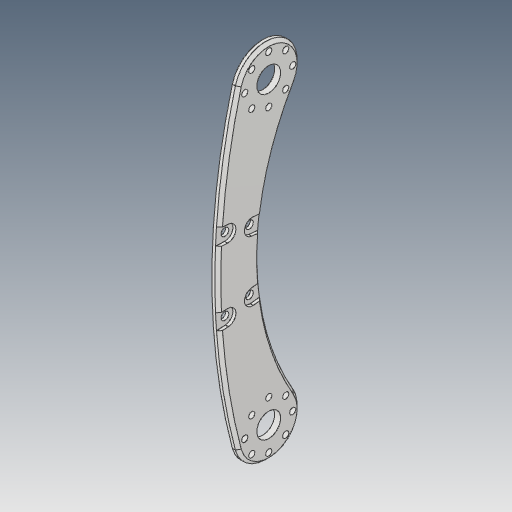
# Autodesk Inventor part: side_frame
Saved by Autodesk Inventor 2019.4 (Build 234330000, 330)
## iProperties
Created: 2018-08-09
Part Number: side_frame
Material: アルミニウム 6061
Document SubType Name: Modeling
Designer: student
Density: 2.7 g/cm^3
Appearance: 滑らか - 白
Mass: 9.43005 g
Surface Area: 44.7876 cm^2
Volume: 3.49261 cm^3
Author: student
Autodesk Inventor part; units mm, degrees
ref_plane "YZ Plane" through (0, 0, 0) normal (1, 0, 0) x (0, 1, 0)
ref_plane "XZ Plane" through (0, 0, 0) normal (0, 1, 0) x (-1, 0, 0)
ref_plane "XY Plane" through (0, 0, 0) normal (0, 0, 1) x (1, 0, 0)
sketch "スケッチ1" plane through (0, 0, 0) normal (1, 0, 0) x (0, 1, 0)
  line L0 (-50, 0) -> (50, 0) construction
  circle A0 centre (-50, 0) radius 4
  circle A1 centre (-50, 0) radius 8 construction
  circle A2 centre (-50, 8) radius 1.05
  line L1 (-50, 8) -> (-50, 0) construction
  circle A3 centre (-55.6569, 5.6569) radius 1.05
  circle A4 centre (-58, 0) radius 1.05
  circle A5 centre (-55.6569, -5.6569) radius 1.05
  circle A6 centre (-50, -8) radius 1.05
  circle A7 centre (-44.3431, -5.6569) radius 1.05
  circle A8 centre (-42, 0) radius 1.05
  circle A9 centre (-44.3431, 5.6569) radius 1.05
  arc A10 (-52.6846, 10.151) -> (-44.7153, -9.0731) centre (-50, 0) ccw
  arc A11 (44.7153, -9.0731) -> (-44.7153, -9.0731) centre (0, -85.8426) ccw
  arc A12 (52.6846, 10.151) -> (-52.6846, 10.151) centre (0, -189.0577) ccw
  arc A13 (44.7153, -9.0731) -> (52.6846, 10.151) centre (50, 0) ccw
  circle A14 centre (50, 0) radius 4
  circle A15 centre (50, 0) radius 8 construction
  line L2 (50, 0) -> (50, 8) construction
  circle A16 centre (50, 8) radius 1.05
  circle A17 centre (44.3431, 5.6569) radius 1.05
  circle A18 centre (42, 0) radius 1.05
  circle A19 centre (44.3431, -5.6569) radius 1.05
  circle A20 centre (50, -8) radius 1.05
  circle A21 centre (55.6569, -5.6569) radius 1.05
  circle A22 centre (58, 0) radius 1.05
  circle A23 centre (55.6569, 5.6569) radius 1.05
  line L3 (12.1598, 13.6356) -> (10.1472, 5.4377) construction
  circle A24 centre (12.1598, 13.6356) radius 1.3
  circle A25 centre (10.1472, 5.4377) radius 1.3
  circle A26 centre (12.1598, 13.6356) radius 3 construction
  circle A27 centre (10.1472, 5.4377) radius 3 construction
  circle A28 centre (-12.1598, 13.6356) radius 1.3
  circle A29 centre (-10.1472, 5.4377) radius 1.3
  line L4 (0, 3) -> (0, 0) construction
  line L5 (0, 17) -> (0, 3) construction
  line L6 (-12.1598, 13.6356) -> (-10.1472, 5.4377) construction
  circle A30 centre (-12.1598, 13.6356) radius 3 construction
  circle A31 centre (-10.1472, 5.4377) radius 3 construction
  line L7 (-50, 0) -> (-11.1535, 9.5367) construction
  line L8 (11.1535, 9.5367) -> (50, 0) construction
  dimension "d1" = 16
  dimension "d0" = 8
  dimension "d2" = 2.1
  dimension "d5" = 360
  dimension "d7" = 100
  dimension "d8" = 10.5
  dimension "d9" = 2.1
  dimension "d12" = 360
  dimension "d14" = 3
  dimension "d16" = 2.6
  dimension "d17" = 6
  dimension "d30" = 14
  dimension "d35" = 40
  dimension "d41" = 40
  constraints: 30 centre point, 18 end point, 13 coincident, 11 point on circle, 8 equal radius, 8 tangent, 3 midpoint, 2 perpendicular, 2 vertical, 2 vertical alignment, 1 collinear, 1 horizontal, 39 other
  measures "d0" diameter of A0
  measures "d2" diameter of A2
  measures "d7" distance of L0.start L0.end
  measures "d8" radius of A10
  measures "d9" diameter of A16
  measures "d14" distance from line of L0 L4.start
  measures "d16" diameter of A25
  measures "d17" diameter of A27
  measures "d30" distance of L5.start L4.start
  measures "d35" distance of L7.start L7.end
  measures "d41" distance of L8.start L2.start
extrude "押し出し1" add sketch "スケッチ1" along normal blind 2
chamfer "面取り1" distance 1 angle 45 4 edges at (2, 0, 17) (2, -59.6996, -4.021) (2, 0, 3) (2, 59.6996, -4.021)
sketch "スケッチ2" plane through (2, 0, 0) normal (1, 0, 0) x (0, 0, -1)
  circle A0 centre (-13.6356, -12.1598) radius 1.3 construction
  circle A1 centre (-5.4377, -10.1472) radius 1.3 construction
  arc A2 (9.0731, 44.7153) -> (9.0731, -44.7153) centre (85.8426, 0) ccw construction
  arc A3 (-10.151, 52.6846) -> (-10.151, -52.6846) centre (189.0577, 0) ccw construction
  line L0 (-5.4377, -10.1472) -> (85.8426, 0) construction
  line L1 (-13.6356, -12.1598) -> (189.0577, 0) construction
  line L2 (-13.6356, -12.1598) -> (-16.6302, -12.3394) construction
  arc A4 (-13.4739, -14.8549) -> (-13.7973, -9.4646) centre (-13.6356, -12.1598) ccw
  arc A5 (-5.736, -7.4637) -> (-5.1394, -12.8307) centre (-5.4377, -10.1472) ccw
  line L3 (-5.1394, -12.8307) -> (-2.117, -12.4947)
  line L4 (-5.736, -7.4637) -> (-2.7136, -7.1277)
  line L5 (-13.7973, -9.4646) -> (-16.7742, -9.6432)
  line L6 (-13.4739, -14.8549) -> (-16.4509, -15.0335)
  arc A6 (-16.7742, -9.6432) -> (-16.4509, -15.0335) centre (189.0577, 0) ccw
  arc A7 (-2.7136, -7.1277) -> (-2.117, -12.4947) centre (85.8426, 0) ccw
  arc A8 (-13.7973, 9.4646) -> (-13.4739, 14.8549) centre (-13.6356, 12.1598) ccw
  arc A9 (-5.1394, 12.8307) -> (-5.736, 7.4637) centre (-5.4377, 10.1472) ccw
  line L7 (-5.1394, 12.8307) -> (-2.117, 12.4947)
  line L8 (-5.736, 7.4637) -> (-2.7136, 7.1277)
  line L9 (-13.7973, 9.4646) -> (-16.7742, 9.6432)
  line L10 (-13.4739, 14.8549) -> (-16.4509, 15.0335)
  arc A10 (-16.4509, 15.0335) -> (-16.7742, 9.6432) centre (189.0577, 0) ccw
  arc A11 (-2.117, 12.4947) -> (-2.7136, 7.1277) centre (85.8426, 0) ccw
  circle A12 centre (-5.4377, 10.1472) radius 1.3 construction
  circle A13 centre (-13.6356, 12.1598) radius 1.3 construction
  line L11 (-13.6356, 12.1598) -> (189.0577, 0) construction
  line L12 (85.8426, 0) -> (-5.4377, 10.1472) construction
  point P0 (0, 0)
  dimension "d25" = 5.4
  constraints: 26 end point, 21 point on circle, 8 centre point, 8 parallel, 8 tangent, 6 concentric, 5 equal radius, 1 collinear
  measures "d25" distance between parallel lines of L5 L6
extrude "押し出し2" cut sketch "スケッチ2" against normal blind 1
